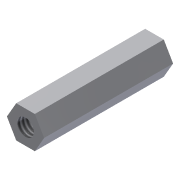
# Autodesk Inventor part: Hex Standoff 8-32 x750
Saved by Autodesk Inventor 2013 (Build 170138000, 138)
## iProperties
Created: 2012-12-09
Part Number: Hex Standoff 8-32 x750
Material: Aluminum 6061
Document SubType Name: Modeling
Designer: Nemo
Density: 2.71 g/cm^3
Mass: 1.36069 g
Surface Area: 6.69374 cm^2
Volume: 0.5021 cm^3
Author: Nemo
Autodesk Inventor part; units mm, degrees
ref_plane "YZ Plane" through (0, 0, 0) normal (1, 0, 0) x (0, 1, 0)
ref_plane "XZ Plane" through (0, 0, 0) normal (0, 1, 0) x (-1, 0, 0)
ref_plane "XY Plane" through (0, 0, 0) normal (0, 0, 1) x (1, 0, 0)
sketch "Sketch1" plane through (0, 0, 0) normal (0, 0, 1) x (1, 0, 0)
  line L0 (-3.6662, 0) -> (-1.8331, 3.175)
  line L1 (-1.8331, 3.175) -> (1.8331, 3.175)
  line L2 (1.8331, 3.175) -> (3.6662, 0)
  line L3 (3.6662, 0) -> (1.8331, -3.175)
  line L4 (1.8331, -3.175) -> (-1.8331, -3.175)
  line L5 (-1.8331, -3.175) -> (-3.6662, 0)
  point P0 (0, 0)
  point P1 (0, 0)
  dimension "d0" = 6.35
  constraints: 12 end point, 1 coincident, 1 horizontal, 13 other
  measures "d0" distance between parallel lines of L4 L1
extrude "Extrusion1" add sketch "Sketch1" along normal mid plane 25.4
sketch "Sketch2" plane through (0, 0, 12.7) normal (0, 0, 1) x (1, 0, 0)
  point P0 (0, 0)
hole "Hole1" at (0, 0, 12.7) direction (0, 0, -1) diameter 3.302 depth 9.525 thread size "8-32 UNC" class "2B" standard "ANSI Unified Screw Threads"
mirror "Mirror1" about plane through (0, 0, 0) normal (0, 0, 1) of "Hole1"
body "Solid1"
